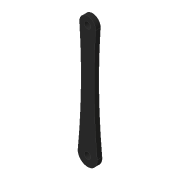
# Autodesk Inventor part: COXA_ROLL_LONG-LINK
Saved by Autodesk Inventor 2019.4 (Build 234330000, 330)
## iProperties
Created: 2019-10-21
Part Number: COXA_ROLL_LONG-LINK
Material: 一般
Document SubType Name: Modeling
Designer: y6tada
Density: 1 g/cm^3
Appearance: Black 60
Author: y6tada
Autodesk Inventor part; units mm, degrees
ref_plane "YZ Plane" through (0, 0, 0) normal (1, 0, 0) x (0, 1, 0)
ref_plane "XZ Plane" through (0, 0, 0) normal (0, 1, 0) x (-1, 0, 0)
ref_plane "XY Plane" through (0, 0, 0) normal (0, 0, 1) x (1, 0, 0)
sketch "スケッチ1" plane through (0, 0, 0) normal (0, 0, 1) x (1, 0, 0)
  line L0 (0, 0) -> (0, -70) construction
  arc A0 (0, -5) -> (4.9881, -0.3446) centre (0, 0) ccw construction
  arc A1 (0, -64) -> (-5.9715, -69.4162) centre (0, -70) ccw construction
  arc A2 (-5.9715, -69.4162) -> (-4.9881, -0.3446) centre (-419.5607, -28.9848) ccw
  arc A3 (4.9881, -0.3446) -> (5.9715, -69.4162) centre (419.5607, -28.9848) ccw
  arc A4 (-4.9881, -0.3446) -> (0, -5) centre (0, 0) ccw construction
  arc A5 (4.9881, -0.3446) -> (-4.9881, -0.3446) centre (0, 0) ccw
  arc A6 (5.9715, -69.4162) -> (0, -64) centre (0, -70) ccw construction
  arc A7 (-5.9715, -69.4162) -> (5.9715, -69.4162) centre (0, -70) ccw
  line L1 (4, 0) -> (4, -70) construction
  dimension "d0" = 70
  dimension "d1" = 5
  dimension "d2" = 6
  dimension "d4" = 4
  constraints: 16 point on circle, 8 centre point, 5 tangent, 4 coincident, 4 end point, 2 point on line, 1 equal radius, 1 parallel, 1 vertical
  measures "d0" distance of L0.start L0.end
  measures "d1" radius of A5
  measures "d2" radius of A7
  measures "d4" distance between parallel lines of L1 L0
extrude "押し出し1" add sketch "スケッチ1" along normal blind 3
hole "穴1" at (0, 0, 0) at (0, -70, 0) direction (0, 0, 1) diameter 4 end through all
